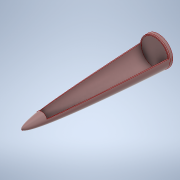
# Autodesk Inventor part: nose-basepart1
Saved by Autodesk Inventor 2020.3 (Build 243373000, 373)
## iProperties
Created: 2021-03-10
Part Number: nose-basepart1
Material: ABS Plastic
Document SubType Name: Modeling
Designer: 0x6f736f646f
Density: 1.06 g/cm^3
Appearance: Smooth - Red
Mass: 17.0739 g
Surface Area: 229.369 cm^2
Volume: 17.0739 cm^3
Author: 0x6f736f646f
Autodesk Inventor part; units mm, degrees
ref_plane "YZ Plane" through (0, 0, 0) normal (1, 0, 0) x (0, 1, 0)
ref_plane "XZ Plane" through (0, 0, 0) normal (0, 1, 0) x (-1, 0, 0)
ref_plane "XY Plane" through (0, 0, 0) normal (0, 0, 1) x (1, 0, 0)
sketch "Sketch2" plane through (0, 0, 0) normal (1, 0, 0) x (0, 1, 0)
  line L0 (0, 0) -> (25.9, 0)
  line L1 (25.9, 0) -> (25.9, -5)
  line L2 (25.9, -5) -> (26.8, -5)
  line L3 (26.8, -5) -> (26.8, 0)
  line L4 (0, 2) -> (25, 2)
  line L5 (0, 0) -> (-25.9, 0)
  line L6 (-25.9, 0) -> (-25.9, -5)
  line L7 (-25.9, -5) -> (-26.8, -5)
  line L8 (-26.8, -5) -> (-26.8, 0)
  line L9 (0, 2) -> (-25, 2)
  line L10 (0, 0) -> (0, 212.5)
  line L11 (0, 0) -> (0, 250)
  line L12 (25, 2) -> (25, 0)
  line L13 (-25, 2) -> (-25, 0)
  line L14 (0, 0) -> (0, 248.2)
  spline S0 degree 2 poles (26.8, 0) (0, 500) (-26.8, 0) knots 0 0 0 1 1 1
  spline S1 degree 2 poles (25, 0) (0, 496.4) (-25, 0) knots 0 0 0 1 1 1
  line L15 (0, 212.5) -> (10.3796, 212.5)
  line L16 (0, 2) -> (-7.0238, 2)
  line L17 (0, 172) -> (0, 2)
  line L18 (0, 214.5) -> (10.099, 214.5)
  line L19 (0, 0) -> (-5, 0)
  line L20 (-5, 0) -> (-5, 212.5)
  line L21 (-5, 212.5) -> (0, 212.5)
  line L22 (0, 212.5) -> (0, 0)
  line L23 (-7.0238, 2) -> (-15.0238, 2)
  line L24 (-15.0238, 2) -> (-5, 212.5)
  line L25 (25, 2) -> (26.6926, 2)
  line L26 (-25, 2) -> (-26.6926, 2)
  line L27 (0, -56.5) -> (0, 304) projected
  line L28 (3, 212.5) -> (3, 2)
  point P0 (24.8991, 2)
  point P1 (9.212, 214.5)
  point P2 (0, 214.5)
  point P3 (9.4814, 212.5)
  dimension "d51" = 25.9
  dimension "d52" = 5
  dimension "d53" = 0.9
  dimension "d54" = 2
  dimension "d55" = 25.9
  dimension "d56" = 5
  dimension "d57" = 0.9
  dimension "d58" = 212.5
  dimension "d59" = 250
  dimension "d60" = 25
  dimension "d61" = 25
  dimension "d62" = 248.2
  dimension "d64" = 25
  dimension "d67" = 2
  dimension "d68" = 212.5
  dimension "d69" = 5
  dimension "d70" = 8
  dimension "d71" = 212.5
  dimension "d72" = 87.274
  dimension "d76" = 3
  constraints: 56 end point, 12 perpendicular, 11 point on line, 8 horizontal, 2 parallel, 1 vertical, 10 other
  measures "d51" distance of L0.start L0.end
  measures "d52" distance of L0.end L1.end
  measures "d53" distance of L1.end L2.end
  measures "d54" distance between parallel lines of L0 L4
  measures "d55" distance of L0.start L5.end
  measures "d56" distance of L5.end L6.end
  measures "d57" distance of L6.end L7.end
  measures "d58" distance of L0.start L10.end
  measures "d59" distance of L0.start L11.end
  measures "d60" distance of L4.start L4.end
  measures "d61" distance of L4.start L9.end
  measures "d62" distance of L0.start L14.end
  measures "d64" distance between parallel lines of L10 L12
  measures "d67" distance between parallel lines of L15 L18
  measures "d68" distance between parallel lines of L0 L15
  measures "d69" distance of L20.end L21.end
  measures "d70" distance of L16.end L23.end
  measures "d71" distance of L19.end L20.end
  measures "d72" angle of L23 L24
  measures "d76" distance between parallel lines of L14 L28
revolve "Revolution5" add sketch "Sketch2" angle 360 mid plane about axis through (0, 0, -10) along (0, 0, 1) contours L10 L4 S1 L0 | L12 L25 S0 L3 L2 L1 L0 | L4 S1 L15 S0 L25 | S1 L18 S0 L15 | S1 L11 S0 L18
extrude "Extrusion4" cut sketch "Sketch2" along normal mid plane 60 contours L4 S1 L15 S0 L25 | L4 L28 L15 S1
sketch "Sketch3" plane through (0, 0, 0) normal (0, 1, 0) x (-1, 0, 0)
  circle A0 centre (0, 102.5) radius 2.5
  point P0 (0, 0)
  dimension "d77" = 5
  constraints: 1 centre point
  measures "d77" diameter of A0
extrude "Extrusion5" cut sketch "Sketch3" against normal blind 30
body "Solid4"
